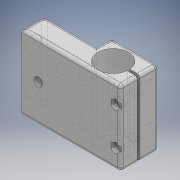
# Autodesk Inventor part: CarroXY - Extrusor V2
Saved by Autodesk Inventor 2017 (Build 210142000, 142)
## iProperties
Created: 2020-08-12
Part Number: CarroXY - Extrusor V2
Material: Generic
Document SubType Name: Modeling
Designer: ale
Density: 1 g/cm^3
Appearance: Default
Author: ale
Autodesk Inventor part; units mm, degrees
ref_plane "YZ Plane" through (0, 0, 0) normal (1, 0, 0) x (0, 1, 0)
ref_plane "XZ Plane" through (0, 0, 0) normal (0, 1, 0) x (-1, 0, 0)
ref_plane "XY Plane" through (0, 0, 0) normal (0, 0, 1) x (1, 0, 0)
sketch "Sketch1" plane through (0, 0, 0) normal (0, 0, 1) x (1, 0, 0)
  arc A0 (10.2228, 0.7464) -> (10.2114, -0.8882) centre (0, 0) ccw
  line L0 (17, -12) -> (-49, -12)
  line L1 (-49, -12) -> (-49, 13)
  line L2 (-49, 13) -> (17, 13)
  line L3 (10.2228, 0.7464) -> (17, 0.7464)
  line L4 (10.2114, -0.8882) -> (17, -0.8882)
  line L5 (17, 13) -> (17, 0.7464)
  line L6 (17, -0.8882) -> (17, -12)
  dimension "d0" = 20.5
  dimension "d1" = 12
  dimension "d2" = 25
  dimension "d4" = 49
  dimension "d33" = 17
  dimension "d34" = 17
  constraints: 14 end point, 3 parallel, 2 point on circle, 1 centre point, 1 coincident, 1 horizontal, 1 perpendicular
  measures "d0" diameter of A0
  measures "d1" distance from line of L0 point (0, 0)
  measures "d2" distance between parallel lines of L2 L0
  measures "d4" distance from line of L1 point (0, 0)
  measures "d33" distance from line of L5 point (0, 0)
  measures "d34" distance from line of L6 point (0, 0)
extrude "Extrusion1" add sketch "Sketch1" along normal blind 50
sketch "Sketch2" plane through (0, 0, 50) normal (0, 0, 1) x (1, 0, 0)
  line L0 (17, 13) -> (-49, 13) projected
  line L1 (-49, 13) -> (-14, 13)
  line L2 (-14, 13) -> (-14, 3)
  line L3 (-14, 3) -> (-49, 3)
  line L4 (-49, 3) -> (-49, 13)
  point P0 (0, 0)
  dimension "d8" = 35
  dimension "d9" = 10
  constraints: 8 end point, 2 parallel, 1 horizontal, 1 perpendicular
  measures "d8" distance of L2.end L3.end
  measures "d9" distance of L1.end L2.end
extrude "Extrusion2" cut sketch "Sketch2" against normal through all
sketch "Sketch3" plane through (-49, -12, 0) normal (-1, 0, 0) x (0, 0, 1)
  line L0 (0, 0) -> (50, 0) projected
  line L1 (0, 0) -> (0, 12) projected
  point P0 (12.5, 7.5)
  point P1 (37.5, 7.5)
  dimension "d12" = 7.5
  dimension "d13" = 7.5
  dimension "d14" = 12.5
  dimension "d15" = 12.5
  measures "d12" distance from line of L0 point (12.5, 7.5)
  measures "d13" distance from line of L0 point (37.5, 7.5)
  measures "d14" distance from line of L1 point (12.5, 7.5)
  measures "d15" horizontal distance of L0.end point (37.5, 7.5)
hole "Hole1" at (-49, -4.5, 12.5) at (-49, -4.5, 37.5) direction (1, 0, 0) diameter 10.7 depth 36
sketch "Sketch4" plane through (-49, 3, 50) normal (0, 1, 0) x (1, 0, 0)
  circle A0 centre (11, 25) radius 10
  line L0 (0, 50) -> (35, 50) projected
  line L1 (35, 50) -> (35, 0) projected
  point P0 (49, 50)
  point P1 (30.1466, 50)
  dimension "d23" = 20
  dimension "d24" = 25
  dimension "d25" = 24
  constraints: 1 centre point
  measures "d23" diameter of A0
  measures "d24" distance from line of A0.centre L0
  measures "d25" distance from line of L1 A0.centre
hole "Hole2" at (-38, 3, 25) direction (0, -1, 0) diameter 5.7 end through all
sketch "Sketch5" plane through (17, 13, 50) normal (0, 1, 0) x (1, 0, 0)
  line L0 (0, 0) -> (-31, 0) projected
  line L1 (-31, 50) -> (0, 50) projected
  line L2 (0, 50) -> (0, 0) projected
  point P0 (-17, 50)
  point P1 (-3.35, 12.5)
  point P2 (-3.35, 37.5)
  dimension "d35" = 12.5
  dimension "d36" = 12.5
  dimension "d37" = 3.35
  dimension "d38" = 3.35
  measures "d35" distance from line of L0 point (-3.35, 12.5)
  measures "d36" distance from line of L1 point (-3.35, 37.5)
  measures "d37" distance from line of L2 point (-3.35, 37.5)
  measures "d38" distance from line of L2 point (-3.35, 12.5)
hole "Hole3" at (13.65, 13, 37.5) at (13.65, 13, 12.5) direction (0, -1, 0) diameter 4.5 end through all
sketch "Sketch6" plane through (-49, -12, 0) normal (0, -1, 0) x (1, 0, 0)
  circle A0 centre (62.65, 37.5) radius 2.25 projected
  line L0 (62.65, 34) -> (59.6189, 35.75)
  line L1 (59.6189, 35.75) -> (59.6189, 39.25)
  line L2 (59.6189, 39.25) -> (62.65, 41)
  line L3 (62.65, 41) -> (65.6811, 39.25)
  line L4 (65.6811, 39.25) -> (65.6811, 35.75)
  line L5 (65.6811, 35.75) -> (62.65, 34)
  circle A1 centre (62.65, 12.5) radius 2.25 projected
  line L6 (62.65, 9) -> (59.6189, 10.75)
  line L7 (59.6189, 10.75) -> (59.6189, 14.25)
  line L8 (59.6189, 14.25) -> (62.65, 16)
  line L9 (62.65, 16) -> (65.6811, 14.25)
  line L10 (65.6811, 14.25) -> (65.6811, 10.75)
  line L11 (65.6811, 10.75) -> (62.65, 9)
  point P0 (49, 0)
  dimension "d46" = 7
  dimension "d47" = 7
  constraints: 24 end point, 2 coincident, 26 other
  measures "d46" distance of L0.start L2.end
  measures "d47" distance of L6.start L8.end
extrude "Extrusion3" cut sketch "Sketch6" against normal blind 3
fillet "Fillet1" radius 2 18 edges at (-14, 13, 25) (-49, 3, 25) (-14, 8, 0) (-31.5, 3, 0) (-49, -4.5, 50) (-14, 8, 50) (-31.5, 3, 50) (1.5, 13, 50) (17, 6.8732, 50) (17, -6.4441, 50) (-16, -12, 50) (17, 6.8732, 0) (1.5, 13, 0) (17, 13, 25) (17, -12, 25) (17, -6.4441, 0) (-16, -12, 0) (-49, -4.5, 0)
body "Solid1"
